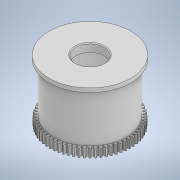
# Autodesk Inventor part: wheel_v6
Saved by Autodesk Inventor 2022 (Build 260153000, 153)
## iProperties
Created: 2022-07-22
Part Number: wheel_v6
Material: 一般
Document SubType Name: Modeling
Designer: Yazawa
Density: 1 g/cm^3
Appearance: 既定
Author: Yazawa
Autodesk Inventor part; units mm, degrees
ref_plane "YZ Plane" through (0, 0, 0) normal (1, 0, 0) x (0, 1, 0)
ref_plane "XZ Plane" through (0, 0, 0) normal (0, 1, 0) x (-1, 0, 0)
ref_plane "XY Plane" through (0, 0, 0) normal (0, 0, 1) x (1, 0, 0)
sketch "スケッチ1" plane through (0, 0, 0) normal (0, 1, 0) x (-1, 0, 0)
  circle A0 centre (0, 0) radius 8
  circle A1 centre (0, 0) radius 9
  circle A2 centre (0, 0) radius 9.9
  circle A3 centre (0, 0) radius 3.5
  dimension "d0" = 16
  dimension "d1" = 18
  dimension "d2" = 19.8
  dimension "d3" = 7
  constraints: 4 centre point, 4 coincident
  measures "d0" diameter of A0
  measures "d1" diameter of A1
  measures "d2" diameter of A2
  measures "d3" diameter of A3
extrude "押し出し1" add sketch "スケッチ1" along normal blind 14 contours A0 | A1 | A3
sketch "スケッチ2" plane through (0, 0, 0) normal (0, -1, 0) x (1, 0, 0)
  circle A0 centre (0, 0) radius 10
  dimension "d6" = 20
  constraints: 1 centre point, 1 coincident
  measures "d6" diameter of A0
extrude "押し出し2" add sketch "スケッチ2" against normal blind 2
sketch "スケッチ3" plane through (0, 14, 0) normal (0, 1, 0) x (1, 0, 0)
  circle A0 centre (0, 0) radius 8
  dimension "d9" = 16
  constraints: 1 centre point, 1 coincident
  measures "d9" diameter of A0
extrude "押し出し3" cut sketch "スケッチ3" along normal up to surface (12 mm away) from surface at -12
sketch "スケッチ4" plane through (0, 2, 0) normal (0, 1, 0) x (1, 0, 0)
  circle A0 centre (0, 0) radius 3.5
  dimension "d12" = 7
  constraints: 1 centre point, 1 coincident
  measures "d12" diameter of A0
extrude "押し出し4" cut sketch "スケッチ4" against normal blind 10
chamfer "面取り1" distance 0.2 angle 45 1 edges at (-3.5, 0, 0)
sketch "スケッチ5" plane through (0, 14, 0) normal (0, 1, 0) x (1, 0, 0)
  circle A0 centre (0, 0) radius 10
  dimension "d18" = 20
  constraints: 1 centre point, 1 coincident
  measures "d18" diameter of A0
extrude "押し出し5" add sketch "スケッチ5" along normal blind 1
sketch "スケッチ8" plane through (0, 15, 0) normal (0, 1, 0) x (1, 0, 0)
  circle A0 centre (0, 0) radius 8 projected
extrude "押し出し8" add sketch "スケッチ8" against normal blind 2
sketch "スケッチ9" plane through (0, 15, 0) normal (0, 1, 0) x (1, 0, 0)
  circle A0 centre (0, 0) radius 3.5
  dimension "d32" = 7
  constraints: 1 centre point, 1 coincident
  measures "d32" diameter of A0
extrude "押し出し9" cut sketch "スケッチ9" against normal blind 2
chamfer "面取り3" distance 0.2 angle 45 1 edges at (-3.5, 15, 0)
sketch "スケッチ10" plane through (0, 2, 0) normal (0, 1, 0) x (1, 0, 0)
  circle A0 centre (0, 0) radius 8 projected
  circle A1 centre (0, 0) radius 3.5 projected
extrude "押し出し10" add sketch "スケッチ10" along normal blind 3 from surface at -2
sketch "スケッチ11" plane through (0, 0, 0) normal (0, -1, 0) x (1, 0, 0)
  circle A0 centre (0, 0) radius 4.5
  dimension "d40" = 9
  constraints: 1 centre point, 1 coincident
  measures "d40" diameter of A0
extrude "押し出し11" cut sketch "スケッチ11" against normal blind 1
chamfer "面取り4" distance 0.2 angle 45 1 edges at (-3.5, 1, 0)
spur gear teeth "平歯車1" teeth 64 pitch diameter 19.2 tip diameter 19.8009 root diameter 18.4509 face width 2 trims to tip circle yes start plane through (0, 0, 0) normal (0, -1, 0) x (1, 0, 0)
